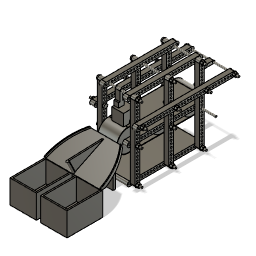
Конвеер v3 (Autodesk Fusion 360 design; units mm, degrees)
Autodesk Fusion 360 part; units mm, degrees
note: some values were not read from the file. Set by a fixed rule: which sketch regions a step uses.
box "BoxPrimitive1" add length 25 width 25 height 25 placed x (0, 0, 1) y (1, 0, 0) z (0, 1, 0) at (0, 0, 0) makes body 1
sketch "Sketch2" plane through (0, 0, 0) normal (0, 1, 0) x (1, 0, 0)
  line L0 (0, 0) -> (-70, 0)
  line L1 (-70, 0) -> (-70, -50)
  line L2 (-70, -50) -> (0, -50)
  line L3 (0, -50) -> (0, 0)
  line L4 (-75, -55) -> (5, -55)
  line L5 (5, -55) -> (5, 5)
  line L6 (5, 5) -> (-75, 5)
  line L7 (-75, 5) -> (-75, -55)
  dimension "d6" = 5
  constraint horizontal L0
  constraint vertical L1
  constraint horizontal L2
  constraint vertical L3
  constraint coincident L0.start L3.end
extrude "Extrude1" add sketch "Sketch2" along normal blind 4 separate body contours L0 L1 L2 L3 makes body 2
extrude "Extrude2" add sketch "Sketch2" along normal blind 50 bodies 2
sketch "Sketch3" plane through (0, 50, 0) normal (0, 1, 0) x (-1, 0, 0)
  line L0 (0, 0) -> (0, 50)
  line L1 (0, 50) -> (70, 50)
  line L2 (70, 50) -> (70, 0)
  line L3 (70, 0) -> (0, 0)
  line L4 (75, -5) -> (75, 55)
  line L5 (75, 55) -> (-5, 55)
  line L6 (-5, 55) -> (-5, -5)
  line L7 (-5, -5) -> (75, -5)
  line L8 (-3, 53) -> (73, 53)
  line L9 (73, 53) -> (73, -3)
  line L10 (73, -3) -> (-3, -3)
  line L11 (-3, -3) -> (-3, 53)
  dimension "d11" = -3
extrude "Extrude3" cut sketch "Sketch3" against normal blind 80 contours L4 L5 L6 L7 bodies 2
sketch "Sketch4" plane through (0, 0, 0) normal (1, 0, 0) x (0, 0, -1)
  line L0 (0, 0) -> (150, 0)
  line L1 (150, 10) -> (0, 10)
  arc A0 (150, 0) -> (150, 10) centre (150, 5) ccw
  arc A1 (0, 10) -> (0, 0) centre (0, 5) ccw
  circle A2 centre (150, 5) radius 2
  circle A3 centre (143.4783, 5) radius 2
  circle A4 centre (136.9565, 5) radius 2
  circle A5 centre (130.4348, 5) radius 2
  circle A6 centre (123.913, 5) radius 2
  circle A7 centre (117.3913, 5) radius 2
  circle A8 centre (110.8696, 5) radius 2
  circle A9 centre (104.3478, 5) radius 2
  circle A10 centre (97.8261, 5) radius 2
  circle A11 centre (91.3043, 5) radius 2
  circle A12 centre (84.7826, 5) radius 2
  circle A13 centre (78.2609, 5) radius 2
  circle A14 centre (71.7391, 5) radius 2
  circle A15 centre (65.2174, 5) radius 2
  circle A16 centre (58.6957, 5) radius 2
  circle A17 centre (52.1739, 5) radius 2
  circle A18 centre (45.6522, 5) radius 2
  circle A19 centre (39.1304, 5) radius 2
  circle A20 centre (32.6087, 5) radius 2
  circle A21 centre (26.087, 5) radius 2
  circle A22 centre (19.5652, 5) radius 2
  circle A23 centre (13.0435, 5) radius 2
  circle A24 centre (6.5217, 5) radius 2
  circle A25 centre (0, 5) radius 2
  dimension "d14" = 4
  dimension "d17" = -150
  dimension "d18" = 0
  constraint horizontal L0
  constraint horizontal L1
  constraint coincident L0.start A1.end
  constraint concentric A0 A2
  measures "d14" diameter of A2
extrude "Extrude4" add sketch "Sketch4" along normal blind 10 separate body makes body 3
sketch "Sketch5" plane through (0, 0, 0) normal (1, 0, 0) x (0, 0, -1)
  circle A0 centre (97.8261, 5) radius 2
  circle A1 centre (26.087, 5) radius 2
  circle A2 centre (32.6087, 5) radius 2
  circle A3 centre (0, 5) radius 2
  circle A4 centre (6.5217, 5) radius 2
  circle A5 centre (13.0435, 5) radius 2
  circle A6 centre (19.5652, 5) radius 2
  circle A7 centre (39.1304, 5) radius 2
  circle A8 centre (65.2174, 5) radius 2
  circle A9 centre (45.6522, 5) radius 2
  circle A10 centre (52.1739, 5) radius 2
  circle A11 centre (71.7391, 5) radius 2
  circle A12 centre (91.3043, 5) radius 2
  circle A13 centre (84.7826, 5) radius 2
  circle A14 centre (78.2609, 5) radius 2
  circle A15 centre (58.6957, 5) radius 2
  circle A16 centre (150, 5) radius 2
  circle A17 centre (136.9565, 5) radius 2
  circle A18 centre (143.4783, 5) radius 2
  circle A19 centre (130.4348, 5) radius 2
  circle A20 centre (110.8696, 5) radius 2
  circle A21 centre (104.3478, 5) radius 2
  circle A22 centre (117.3913, 5) radius 2
  circle A23 centre (123.913, 5) radius 2
  arc A24 (0, 10) -> (0, 0) centre (0, 5) ccw
  line L0 (0, 10) -> (150, 10)
  arc A25 (150, 0) -> (150, 10) centre (150, 5) ccw
  line L1 (150, 0) -> (0, 0)
  circle A26 centre (143.4783, 5) radius 20
  circle A27 centre (143.4783, 5) radius 23
  dimension "d21" = 40
  dimension "d22" = 46
  constraint concentric A18 A26
  constraint concentric A18 A27
  measures "d21" diameter of A26
  measures "d22" diameter of A27
extrude "Extrude5" add sketch "Sketch5" against normal blind 40 separate body contours A16 | A17 | A19 | A23 A26 | A23 L0 A25 L1 A26 | A23 A26 | A23 L0 L1 A26 A27 | L0 A25 L1 A26 | L0 L1 A26 A27 makes body 4
copy_body "CopyPasteBodies1" bodies 3 makes body 5
move_body "Move1" bodies 5 to x (1, 0, 0) y (0, 1, 0) z (0, 0, 1) at (-50, 0, 0)
copy_body "CopyPasteBodies2" bodies 4 makes body 6
move_body "Move2" bodies 6 to x (1, 0, 0) y (0, 1, 0) z (0, 0, 1) at (0, 0, 137)
copy_body "CopyPasteBodies3" bodies 4 makes body 7
move_body "Move3" bodies 7 to x (1, 0, 0) y (0, 1, 0) z (0, 0, 1) at (0, 0, 65)
move_body "Align1" bodies 7 to x (1, 0, 0) y (0, 1, 0) z (0, 0, 1) at (0, 0, 0.2174)
sketch "Sketch6" plane through (-40, 0, 0) normal (-1, 0, 0) x (0, 0, 1)
  circle A0 centre (-143.4783, 5) radius 2
  circle A1 centre (-143.4783, 5) radius 23
  circle A2 centre (-143.4783, 5) radius 23
  circle A3 centre (-78.2609, 5) radius 23
  circle A4 centre (-6.4783, 5) radius 23
  line L0 (-6.4783, 5) -> (-6.4783, 28)
  line L1 (-143.4783, 5) -> (-143.4783, 28)
  line L2 (-143.4783, 28) -> (-6.4783, 28)
  line L3 (-143.4783, 5) -> (-143.4783, -18)
  line L4 (-6.4783, 5) -> (-6.4783, -18)
  line L5 (-6.4783, -18) -> (-143.4783, -18)
  arc A5 (-143.4783, 28) -> (-143.4783, -18) centre (-143.4783, 5) ccw
  arc A6 (-6.4783, -18) -> (-6.4783, 28) centre (-6.4783, 5) ccw
  arc A7 (-143.4783, 29) -> (-143.4783, -19) centre (-143.4783, 5) ccw
  line L6 (-6.4783, -19) -> (-143.4783, -19)
  arc A8 (-6.4783, -19) -> (-6.4783, 29) centre (-6.4783, 5) ccw
  line L7 (-143.4783, 29) -> (-6.4783, 29)
  dimension "d25" = 1
  constraint coincident A4.centre L0.start
  constraint coincident A4 L0.end
  constraint vertical L0
  constraint coincident A0.centre A1.centre
  constraint coincident A2 L1.end
  constraint parallel L0 L1
  constraint coincident A2 L3.end
  constraint perpendicular L2 L3
  constraint coincident A4 L4.end
  constraint parallel L0 L4
  constraint tangent L5 A5
  constraint tangent L2 A6
extrude "Extrude6" add sketch "Sketch6" against normal blind 40 separate body makes body 8
sketch "Sketch7" plane through (0, 0, 0) normal (1, 0, 0) x (0, 0, -1)
  arc A0 (6.4783, 29) -> (6.4783, -19) centre (6.4783, 5) ccw
  line L0 (-20, -19) -> (-90, -19)
  line L1 (-20, 15) -> (-20, -19)
  line L2 (-20, 15) -> (-90, -19)
  constraint tangent A0 L0
  constraint perpendicular L0 L1
extrude "Extrude7" add sketch "Sketch7" against normal blind 40 separate body makes body 9
move_body "Move4" bodies 2 to x (0, 0, -1) y (0, 1, 0) z (1, 0, 0) at (-70, -71, 89)
move_body "Move5" bodies 2 to x (1, 0, 0) y (0, 1, 0) z (0, 0, 1) at (25, 0, 0)
copy_body "CopyPasteBodies4" bodies 5 makes body 10
move_body "Move6" bodies 10 to x (1, 0, 0) y (0, 1, 0) z (0, 0, 1) at (0, -72, 0)
sketch "Sketch8" plane through (-50, 0, 0) normal (-1, 0, 0) x (0, 0, 1)
  circle A0 centre (-97.8261, -67) radius 2
  circle A1 centre (-26.087, -67) radius 2
  circle A2 centre (-32.6087, -67) radius 2
  circle A3 centre (0, -67) radius 2
  circle A4 centre (-6.5217, -67) radius 2
  circle A5 centre (-13.0435, -67) radius 2
  circle A6 centre (-19.5652, -67) radius 2
  circle A7 centre (-39.1304, -67) radius 2
  circle A8 centre (-65.2174, -67) radius 2
  circle A9 centre (-45.6522, -67) radius 2
  circle A10 centre (-52.1739, -67) radius 2
  circle A11 centre (-71.7391, -67) radius 2
  circle A12 centre (-91.3043, -67) radius 2
  circle A13 centre (-84.7826, -67) radius 2
  circle A14 centre (-78.2609, -67) radius 2
  circle A15 centre (-58.6957, -67) radius 2
  circle A16 centre (-150, -67) radius 2
  circle A17 centre (-136.9565, -67) radius 2
  circle A18 centre (-143.4783, -67) radius 2
  circle A19 centre (-130.4348, -67) radius 2
  circle A20 centre (-110.8696, -67) radius 2
  circle A21 centre (-104.3478, -67) radius 2
  circle A22 centre (-117.3913, -67) radius 2
  circle A23 centre (-123.913, -67) radius 2
  arc A24 (0, -72) -> (0, -62) centre (0, -67) ccw
  line L0 (0, -62) -> (-150, -62)
  arc A25 (-150, -62) -> (-150, -72) centre (-150, -67) ccw
  line L1 (-150, -72) -> (0, -72)
  line L2 (-136.9565, -67) -> (-141.9565, -67)
  line L3 (-136.9565, -67) -> (-131.9565, -67)
  arc A26 (-141.9565, -67) -> (-131.9565, -67) centre (-136.9565, -67) ccw
  circle A27 centre (-136.9565, -67) radius 2
  line L4 (-141.9565, -67) -> (-141.9565, 90)
  line L5 (-131.9565, -67) -> (-131.9565, -62)
  line L6 (-131.9565, 90) -> (-131.9565, -62)
  arc A28 (-131.9565, 90) -> (-141.9565, 90) centre (-136.9565, 90) ccw
  circle A29 centre (-136.9565, -60.4583) radius 2
  circle A30 centre (-136.9565, -53.9167) radius 2
  circle A31 centre (-136.9565, -47.375) radius 2
  circle A32 centre (-136.9565, -40.8333) radius 2
  circle A33 centre (-136.9565, -34.2917) radius 2
  circle A34 centre (-136.9565, -27.75) radius 2
  circle A35 centre (-136.9565, -21.2083) radius 2
  circle A36 centre (-136.9565, -14.6667) radius 2
  circle A37 centre (-136.9565, -8.125) radius 2
  circle A38 centre (-136.9565, -1.5833) radius 2
  circle A39 centre (-136.9565, 4.9583) radius 2
  circle A40 centre (-136.9565, 11.5) radius 2
  circle A41 centre (-136.9565, 18.0417) radius 2
  circle A42 centre (-136.9565, 24.5833) radius 2
  circle A43 centre (-136.9565, 31.125) radius 2
  circle A44 centre (-136.9565, 37.6667) radius 2
  circle A45 centre (-136.9565, 44.2083) radius 2
  circle A46 centre (-136.9565, 50.75) radius 2
  circle A47 centre (-136.9565, 57.2917) radius 2
  circle A48 centre (-136.9565, 63.8333) radius 2
  circle A49 centre (-136.9565, 70.375) radius 2
  circle A50 centre (-136.9565, 76.9167) radius 2
  circle A51 centre (-136.9565, 83.4583) radius 2
  circle A52 centre (-136.9565, 90) radius 2
  dimension "d30" = 10
  dimension "d33" = 0
  dimension "d34" = 157
  constraint concentric A17 A26
  constraint tangent L1 A26
  constraint coincident A17.centre L2.start
  constraint horizontal L2
  constraint parallel L2 L3
  constraint tangent A26 L4
  constraint tangent A26 L5
  constraint coincident L0 L5.end
  measures "d30" distance of L4.end L6.start
extrude "Extrude8" add sketch "Sketch8" along normal blind 10 separate body contours A17 A18 A19 L2 L3 A26 A27 | A17 A18 A19 L0 L2 L3 A27 L4 L5 A29 | A19 L3 A26 | A19 L3 L5 | A18 L2 L4 | A18 L2 A26 | L0 L4 L6 A28 A29 makes body 11
copy_body "CopyPasteBodies5" bodies 11 makes body 12
move_body "Move7" bodies 12 to x (1, 0, 0) y (0, 1, 0) z (0, 0, 1) at (0, 0, 131)
move_body "Move8" bodies 12 to x (1, 0, 0) y (0, 1, 0) z (0, 0, 1) at (-50, 0, 0)
move_body "Align2" bodies 12 to x (1, 0, 0) y (0, 1, 0) z (0, 0, 1) at (50, 0, -0.5652)
copy_body "CopyPasteBodies6" bodies 12 makes body 13
move_body "Move9" bodies 13 to x (1, 0, 0) y (0, 1, 0) z (0, 0, 1) at (-56, 0, -72)
move_body "Align3" bodies 13 to x (1, 0, 0) y (0, 1, 0) z (0, 0, 1) at (56, 0, 0.2609)
extrude "Extrude9" add 1 faces at (-40, -71, -73.913) along direction (1, 0, 0) blind 50 separate body on bodies 10 makes body 14
combine "Combine1" operation add target body 14 tool bodies 10
copy_body "CopyPasteBodies7" bodies 13 12 11 makes body 15 makes body 16 makes body 17
move_body "Move10" bodies 15 16 17 to x (1, 0, 0) y (0, 1, 0) z (0, 0, 1) at (70, 0, 0)
copy_body "CopyPasteBodies8" bodies 3 5 makes body 18 makes body 19
move_body "Move11" bodies 18 19 to x (1, 0, 0) y (0, 1, 0) z (0, 0, 1) at (0, 85, 0)
sketch "Sketch9" plane through (-40, 0, 0) normal (-1, 0, 0) x (0, 0, 1)
  line L0 (20, 15) -> (20, -19)
  line L1 (20, -19) -> (90, -19)
  line L2 (90, -19) -> (20, 15)
  line L3 (20, 15) -> (90, -19)
  line L4 (90, -19) -> (103.0246, 7.8154)
  line L5 (103.0246, 7.8154) -> (29.3484, 10.4593)
  constraint coincident L0.start L2.end
  constraint coincident L1.end L2.start
  constraint perpendicular L3 L4
  constraint coincident L2 L5.end
extrude "Extrude10" add sketch "Sketch9" against normal blind 3 separate body contours L2 L3 L4 L5 makes body 20
move_body "Move12" bodies 20 to x (1, 0, 0) y (0, 1, 0) z (0, 0, 1) at (17, 0, 0)
move_body "Move13" bodies 16 to x (1, 0, 0) y (0, 1, 0) z (0, 0, 1) at (60, 0, 0)
move_body "Move14" bodies 15 to x (1, 0, 0) y (0, 1, 0) z (0, 0, 1) at (60, 0, 0)
move_body "Align4" bodies 16 to x (1, 0, 0) y (0, 1, 0) z (0, 0, 1) at (-60, 0, 6.5217)
move_body "Align5" bodies 15 to x (1, 0, 0) y (0, 1, 0) z (0, 0, 1) at (-60, 0, 0)
move_body "Move15" bodies 16 to x (1, 0, 0) y (0, 1, 0) z (0, 0, 1) at (50, 0, 0)
move_body "Align6" bodies 16 to x (1, 0, 0) y (0, 1, 0) z (0, 0, 1) at (-50, 0, -6.5217)
sketch "Sketch10" plane through (20, 0, 0) normal (1, 0, 0) x (0, 0, -1)
  circle A0 centre (6.5217, 50.75) radius 2
  circle A1 centre (6.5217, 57.2917) radius 2
  circle A2 centre (6.5217, 63.8333) radius 2
  circle A3 centre (6.5217, 76.9167) radius 2
  circle A4 centre (6.5217, 4.9583) radius 2
  circle A5 centre (6.5217, 70.375) radius 2
  circle A6 centre (6.5217, 11.5) radius 2
  circle A7 centre (6.5217, 44.2083) radius 2
  circle A8 centre (6.5217, 24.5833) radius 2
  circle A9 centre (6.5217, 31.125) radius 2
  circle A10 centre (6.5217, 37.6667) radius 2
  circle A11 centre (6.5217, 18.0417) radius 2
  circle A12 centre (6.5217, -40.8333) radius 2
  circle A13 centre (6.5217, -47.375) radius 2
  circle A14 centre (6.5217, -53.9167) radius 2
  circle A15 centre (6.5217, -1.5833) radius 2
  circle A16 centre (6.5217, -34.2917) radius 2
  circle A17 centre (6.5217, -27.75) radius 2
  circle A18 centre (6.5217, -21.2083) radius 2
  circle A19 centre (6.5217, -8.125) radius 2
  circle A20 centre (6.5217, -14.6667) radius 2
  circle A21 centre (6.5217, -60.4583) radius 2
  circle A22 centre (6.5217, 83.4583) radius 2
  circle A23 centre (6.5217, -67) radius 2
  circle A24 centre (6.5217, 90) radius 2
  arc A25 (1.5217, -67) -> (11.5217, -67) centre (6.5217, -67) ccw
  line L0 (11.5217, -67) -> (11.5217, 90)
  arc A26 (11.5217, 90) -> (1.5217, 90) centre (6.5217, 90) ccw
  line L1 (1.5217, 90) -> (1.5217, -67)
move_body "Move16" bodies 5 to x (1, 0, 0) y (0, 1, 0) z (0, 0, 1) at (20, 0, 0)
move_body "Align7" bodies 5 to x (1, 0, 0) y (0, 1, 0) z (0, 0, 1) at (-20, -0.0417, 0)
move_body "Move17" bodies 3 to x (1, 0, 0) y (0, 1, 0) z (0, 0, 1) at (-15, 0, 0)
move_body "Align8" bodies 3 to x (1, 0, 0) y (0, 1, 0) z (0, 0, 1) at (15, -0.0417, 0)
move_body "Align9" bodies 5 to x (1, 0, 0) y (0, 1, 0) z (0, 0, 1) at (0, 0.0417, 0.0435)
sketch "Sketch11" plane through (-60, 0, 0) normal (-1, 0, 0) x (0, 0, 1)
  circle A0 centre (-136.9565, 50.75) radius 2
  circle A1 centre (-136.9565, 57.2917) radius 2
  circle A2 centre (-136.9565, 63.8333) radius 2
  circle A3 centre (-136.9565, 76.9167) radius 2
  circle A4 centre (-136.9565, 4.9583) radius 2
  circle A5 centre (-136.9565, 70.375) radius 2
  circle A6 centre (-136.9565, 11.5) radius 2
  circle A7 centre (-136.9565, 44.2083) radius 2
  circle A8 centre (-136.9565, 24.5833) radius 2
  circle A9 centre (-136.9565, 31.125) radius 2
  circle A10 centre (-136.9565, 37.6667) radius 2
  circle A11 centre (-136.9565, 18.0417) radius 2
  circle A12 centre (-136.9565, -40.8333) radius 2
  circle A13 centre (-136.9565, -47.375) radius 2
  circle A14 centre (-136.9565, -53.9167) radius 2
  circle A15 centre (-136.9565, -1.5833) radius 2
  circle A16 centre (-136.9565, -34.2917) radius 2
  circle A17 centre (-136.9565, -27.75) radius 2
  circle A18 centre (-136.9565, -21.2083) radius 2
  circle A19 centre (-136.9565, -8.125) radius 2
  circle A20 centre (-136.9565, -14.6667) radius 2
  circle A21 centre (-136.9565, -60.4583) radius 2
  circle A22 centre (-136.9565, 83.4583) radius 2
  circle A23 centre (-136.9565, -67) radius 2
  circle A24 centre (-136.9565, 90) radius 2
  arc A25 (-141.9565, -67) -> (-131.9565, -67) centre (-136.9565, -67) ccw
  line L0 (-131.9565, -67) -> (-131.9565, 90)
  arc A26 (-131.9565, 90) -> (-141.9565, 90) centre (-136.9565, 90) ccw
  line L1 (-141.9565, 90) -> (-141.9565, -67)
  circle A27 centre (-136.9565, 90) radius 4
  dimension "d41" = 8
  constraint concentric A24 A27
  measures "d41" diameter of A27
extrude "Extrude11" add sketch "Sketch11" against normal blind 90 separate body contours A24 makes body 21
extrude "Extrude12" add sketch "Sketch11" along normal blind 3 separate body contours A24 | A27 makes body 22
combine "Combine2" operation add target body 22 tool bodies 21
copy_body "CopyPasteBodies9" bodies 22 makes body 23
copy_body "CopyPasteBodies10" bodies 23 makes body 24
sketch "Sketch12" plane through (20, 0, 0) normal (1, 0, 0) x (0, 0, -1)
  circle A0 centre (136.9565, 50.75) radius 2
  circle A1 centre (136.9565, 57.2917) radius 2
  circle A2 centre (136.9565, 63.8333) radius 2
  circle A3 centre (136.9565, 76.9167) radius 2
  circle A4 centre (136.9565, 4.9583) radius 2
  circle A5 centre (136.9565, 70.375) radius 2
  circle A6 centre (136.9565, 11.5) radius 2
  circle A7 centre (136.9565, 44.2083) radius 2
  circle A8 centre (136.9565, 24.5833) radius 2
  circle A9 centre (136.9565, 31.125) radius 2
  circle A10 centre (136.9565, 37.6667) radius 2
  circle A11 centre (136.9565, 18.0417) radius 2
  circle A12 centre (136.9565, -40.8333) radius 2
  circle A13 centre (136.9565, -47.375) radius 2
  circle A14 centre (136.9565, -53.9167) radius 2
  circle A15 centre (136.9565, -1.5833) radius 2
  circle A16 centre (136.9565, -34.2917) radius 2
  circle A17 centre (136.9565, -27.75) radius 2
  circle A18 centre (136.9565, -21.2083) radius 2
  circle A19 centre (136.9565, -8.125) radius 2
  circle A20 centre (136.9565, -14.6667) radius 2
  circle A21 centre (136.9565, -60.4583) radius 2
  circle A22 centre (136.9565, 83.4583) radius 2
  circle A23 centre (136.9565, -67) radius 2
  circle A24 centre (136.9565, 90) radius 2
  arc A25 (131.9565, -67) -> (141.9565, -67) centre (136.9565, -67) ccw
  line L0 (141.9565, -67) -> (141.9565, 90)
  arc A26 (141.9565, 90) -> (131.9565, 90) centre (136.9565, 90) ccw
  line L1 (131.9565, 90) -> (131.9565, -67)
  circle A27 centre (136.9565, 90) radius 2
  line L2 (134.9358, 93.5) -> (132.9151, 90)
  line L3 (132.9151, 90) -> (134.9358, 86.5)
  line L4 (134.9358, 86.5) -> (138.9772, 86.5)
  line L5 (138.9772, 86.5) -> (140.998, 90)
  line L6 (140.998, 90) -> (138.9772, 93.5)
  line L7 (138.9772, 93.5) -> (134.9358, 93.5)
  point P0 (136.9565, 90)
  dimension "d46" = 3.5
  constraint coincident P0 A24.centre
  measures "d46" distance of P0 L7
extrude "Extrude13" add sketch "Sketch12" along normal blind 5 separate body contours L2 L3 L4 L5 L6 L7 makes body 25
copy_body "CopyPasteBodies11" bodies 25 24 makes body 26 makes body 27
move_body "Move18" bodies 26 27 to x (1, 0, 0) y (0, 1, 0) z (0, 0, 1) at (0, 0, 59)
copy_body "CopyPasteBodies12" bodies 27 26 makes body 28 makes body 29
move_body "Move19" bodies 28 29 to x (1, 0, 0) y (0, 1, 0) z (0, 0, 1) at (0, 0, 70)
delete_body "RemoveBody2" bodies 23
delete_body "RemoveBody3" bodies 22
move_body "Align10" bodies 17 to x (1, 0, 0) y (0, 1, 0) z (0, 0, 1) at (0, 0, 0)
move_body "Align11" bodies 27 to x (1, 0, 0) y (0, 1, 0) z (0, 0, 1) at (0, 0, -0.3043)
move_body "Align12" bodies 28 to x (1, 0, 0) y (0, 1, 0) z (0, 0, 1) at (0, 0, 1.4348)
move_body "Align13" bodies 26 to x (0, 0, 1) y (0, 1, 0) z (-1, 0, 0) at (-55.4565, 0, -100.7609)
move_body "Align14" bodies 26 to x (0, 0, 1) y (0, 1, 0) z (-1, 0, 0) at (-53.2609, 0, -100.7609)
move_body "Move20" bodies 26 to x (1, 0, 0) y (0, 1, 0) z (0, 0, 1) at (5.5, 0, 0)
move_body "Align15" bodies 26 to x (1, 0, 0) y (0, 1, 0) z (0, 0, 1) at (-8, 0, 0)
move_body "Align16" bodies 29 to x (1, 0, 0) y (0, 1, 0) z (0, 0, 1) at (0, 0, 1.4348)
copy_body "CopyPasteBodies13" bodies 29 28 27 26 25 24 makes body 30 makes body 31 makes body 32 makes body 33 makes body 34 makes body 35
move_body "Move21" bodies 30 31 32 33 34 35 to x (1, 0, 0) y (0, 1, 0) z (0, 0, 1) at (0, -85, 0)
move_body "Align17" bodies 11 to x (1, 0, 0) y (0, 1, 0) z (0, 0, 1) at (0, 0, -6.5217)
move_body "Align18" bodies 17 to x (1, 0, 0) y (0, 1, 0) z (0, 0, 1) at (0, 0, -6.5217)
move_body "Align19" bodies 24 to x (1, 0, 0) y (0, 1, 0) z (0, 0, 1) at (0, 0, -6.5217)
move_body "Align20" bodies 25 to x (1, 0, 0) y (0, 1, 0) z (0, 0, 1) at (0, 0, -6.5217)
move_body "Align21" bodies 35 to x (1, 0, 0) y (0, 1, 0) z (0, 0, 1) at (0, -0.0417, -6.5217)
move_body "Align22" bodies 34 to x (1, 0, 0) y (0, 1, 0) z (0, 0, 1) at (0, -0.0417, -6.5217)
copy_body "CopyPasteBodies14" bodies 35 34 33 32 31 30 makes body 36 makes body 37 makes body 38 makes body 39 makes body 40 makes body 41
move_body "Move22" bodies 36 37 38 39 40 41 to x (1, 0, 0) y (0, 1, 0) z (0, 0, 1) at (0, -72, 0)
move_body "Move23" bodies 20 to x (1, 0, 0) y (0, 1, 0) z (0, 0, 1) at (0, 2.1845, -4.4975)
sketch "Sketch13" plane through (0, 19.9967, 9.7127) normal (0, 0.899508, 0.436904) x (1, 0, 0)
  line L0 (0, -89.2569) -> (0, -11.4366)
  line L1 (0, -11.4366) -> (-40, -11.4366)
  line L2 (-40, -11.4366) -> (-40, -89.2569)
  line L3 (-40, -89.2569) -> (0, -89.2569)
  line L4 (-23, -16.8294) -> (-23, -84.2569)
  line L5 (-23, -84.2569) -> (-20, -84.2569)
  line L6 (-20, -84.2569) -> (-20, -16.8294)
  line L7 (-20, -16.8294) -> (-23, -16.8294)
  line L8 (-23, -84.2569) -> (-23.7059, -85.5804)
  line L9 (-20, -84.2569) -> (-19.2941, -85.5804)
  arc A0 (-23.7059, -85.5804) -> (-19.2941, -85.5804) centre (-21.5, -86.7569) ccw
  constraint tangent L5 A0
  constraint coincident L4.end L5.start
  constraint tangent L8 A0
  constraint coincident L5.end L6.start
  constraint tangent L9 A0
extrude "Extrude14" add sketch "Sketch13" along normal blind 29.9 separate body contours L5 L8 L9 A0 makes body 42
combine "Combine3" operation add target body 20 tool bodies 42
copy_body "CopyPasteBodies15" bodies 2 makes body 43
move_body "Move24" bodies 43 to x (1, 0, 0) y (0, 1, 0) z (0, 0, 1) at (-65, 0, 0)
move_body "Move25" bodies 2 43 to x (1, 0, 0) y (0, 1, 0) z (0, 0, 1) at (31, 0, 0)
sketch "Sketch14" plane through (-40, 0, 0) normal (-1, 0, 0) x (0, 0, 1)
  line L0 (20, 15) -> (20, -19)
  line L1 (20, -19) -> (90, -19)
  line L2 (90, -19) -> (20, 15)
  circle A0 centre (-97.8261, -67) radius 2
  circle A1 centre (-26.087, -67) radius 2
  circle A2 centre (-32.6087, -67) radius 2
  circle A3 centre (0, -67) radius 2
  circle A4 centre (-6.5217, -67) radius 2
  circle A5 centre (-13.0435, -67) radius 2
  circle A6 centre (-19.5652, -67) radius 2
  circle A7 centre (-39.1304, -67) radius 2
  circle A8 centre (-65.2174, -67) radius 2
  circle A9 centre (-45.6522, -67) radius 2
  circle A10 centre (-52.1739, -67) radius 2
  circle A11 centre (-71.7391, -67) radius 2
  circle A12 centre (-91.3043, -67) radius 2
  circle A13 centre (-84.7826, -67) radius 2
  circle A14 centre (-78.2609, -67) radius 2
  circle A15 centre (-58.6957, -67) radius 2
  circle A16 centre (-150, -67) radius 2
  circle A17 centre (-136.9565, -67) radius 2
  circle A18 centre (-143.4783, -67) radius 2
  circle A19 centre (-130.4348, -67) radius 2
  circle A20 centre (-110.8696, -67) radius 2
  circle A21 centre (-104.3478, -67) radius 2
  circle A22 centre (-117.3913, -67) radius 2
  circle A23 centre (-123.913, -67) radius 2
  arc A24 (0, -72) -> (0, -62) centre (0, -67) ccw
  line L3 (0, -62) -> (-150, -62)
  arc A25 (-150, -62) -> (-150, -72) centre (-150, -67) ccw
  line L4 (-150, -72) -> (0, -72)
  line L5 (0, -72) -> (85, -72)
  line L6 (20, -19) -> (20, -72)
  line L7 (20, -72) -> (25, -72)
  line L8 (25, -72) -> (25, -19)
  line L9 (25, -19) -> (70, -19)
  line L10 (70, -19) -> (70, -72)
  line L11 (70, -72) -> (75, -72)
  line L12 (75, -72) -> (75, -19)
  dimension "d51" = 5
  constraint coincident A24.start L4.end
  constraint tangent A24 L5
  constraint coincident L0.end L1.start
  constraint coincident L5 L6.end
  constraint perpendicular L5 L6
  constraint perpendicular L6 L7
  constraint coincident L1 L8.end
  constraint perpendicular L1 L8
  constraint coincident L1 L9.end
  constraint coincident L5 L10.end
  constraint perpendicular L5 L10
  constraint coincident L5 L11.end
  constraint coincident L1 L12.end
  constraint perpendicular L1 L12
  measures "d51" distance of L6.end L7.end
extrude "Extrude15" add sketch "Sketch14" against normal blind 40 separate body contours L1 L5 L6 L7 L8 | L1 L5 L10 L11 L12 makes body 44 at (-26.6667, -54.3333, 25) makes body 45 at (-26.6667, -54.3333, 75)
combine "Combine4" operation add target body 45 tool bodies 44 9
sketch "Sketch15" plane through (0, 0, 0) normal (1, 0, 0) x (0, 0, -1)
  line L0 (-70, -72) -> (-70, -19)
  line L1 (-70, -19) -> (-25, -19)
  line L2 (-25, -19) -> (-25, -72)
  line L3 (-25, -72) -> (-20, -72)
  line L4 (-20, -72) -> (-20, 15)
  line L5 (-20, 15) -> (-90, -19)
  line L6 (-90, -19) -> (-75, -19)
  line L7 (-75, -19) -> (-75, -72)
  line L8 (-75, -72) -> (-70, -72)
  line L9 (-20, 15) -> (-20, 11)
  line L10 (-90, -19) -> (-90, -23)
  line L11 (-90, -23) -> (-20, 11)
  constraint coincident L4.end L5.start
  constraint coincident L4 L9.end
  constraint parallel L4 L9
  constraint coincident L5.end L6.start
  constraint perpendicular L6 L10
extrude "Extrude16" add sketch "Sketch15" along normal blind 40 separate body contours L4 L5 L6 L9 L11 makes body 46
copy_body "CopyPasteBodies16" bodies 46 makes body 47
move_body "Move26" bodies 47 to x (1, 0, 0) y (0, 1, 0) z (0, 0, 1) at (-80, 0, 0)
combine "Combine5" operation add target body 47 tool bodies 45 46
sketch "Sketch16" plane through (0, 19.9967, 9.7127) normal (0, 0.899508, 0.436904) x (1, 0, 0)
  line L0 (-80, -11.4366) -> (-80, -89.2569)
  line L1 (-80, -89.2569) -> (40, -89.2569)
  line L2 (40, -89.2569) -> (40, -11.4366)
  line L3 (40, -11.4366) -> (-80, -11.4366)
  arc A0 (-53.5072, -11.4366) -> (-80, -89.2569) centre (47.5418, -89.2569) ccw
  line L4 (-23, -16.8294) -> (-20, -16.8294)
  line L5 (-20, -89.2569) -> (-20, -80)
  arc A1 (40, -89.2569) -> (13.5072, -11.4366) centre (-87.5418, -89.2569) ccw
  constraint tangent L0 A0
  constraint coincident L3 A0.start
  constraint coincident L0.end L1.start
  constraint midpoint L1 L5.start
  constraint perpendicular L1 L5
  constraint symmetric L0.end L5 L1.end
  constraint symmetric A0.start L5 A1.end
  constraint symmetric A0 L5 A1
extrude "Extrude17" cut sketch "Sketch16" against normal blind 5 contours L0 L3 A0 | L2 L3 A1 bodies 43 47
sketch "Sketch17" plane through (0, 19.9967, 9.7127) normal (0, 0.899508, 0.436904) x (1, 0, 0)
  arc A0 (-53.5072, -11.4366) -> (-80, -89.2569) centre (47.5418, -89.2569) ccw
  line L0 (-80, -89.2569) -> (40, -89.2569)
  arc A1 (40, -89.2569) -> (13.5072, -11.4366) centre (-87.5418, -89.2569) ccw
  line L1 (13.5072, -11.4366) -> (-53.5072, -11.4366)
  line L2 (-80, -89.2569) -> (-78, -89.2569)
  line L3 (40, -89.2569) -> (38, -89.2569)
  line L4 (13.5072, -11.4366) -> (11.5072, -11.4366)
  line L5 (-53.5072, -11.4366) -> (-51.5072, -11.4366)
  arc A2 (-51.5072, -11.4366) -> (-78, -89.2569) centre (48.5107, -88.9059) ccw
  arc A3 (38, -89.2569) -> (11.5072, -11.4366) centre (-88.5107, -88.9059) ccw
  dimension "d58" = 2
  dimension "d59" = 2
  dimension "d60" = 2
  constraint coincident A0.end L0.start
  constraint parallel L0 L2
  constraint coincident L0.end A1.start
  constraint coincident L0 L3.end
  constraint parallel L0 L3
  constraint coincident A1.end L1.start
  constraint parallel L1 L4
  constraint coincident A0.start L1.end
  constraint parallel L1 L5
  constraint tangent A0 A2
  constraint tangent A1 A3
  measures "d58" distance of A0.end L2.end
  measures "d59" distance of A1.end L4.end
  measures "d60" distance of A0.start L5.end
extrude "Extrude18" add sketch "Sketch17" along normal blind 4 separate body contours A0 L0 L1 L2 L5 A2 | L0 A1 L1 L3 L4 A3 makes body 48 at (-76.0966, -6.8948, 71.1811) makes body 49 at (37.5387, -11.7297, 81.1353)
combine "Combine6" operation add target body 49 tool bodies 47 48
sketch "Sketch18" plane through (30, 0, 0) normal (1, 0, 0) x (0, 0, -1)
  circle A0 centre (6.5217, 90) radius 2
  circle A1 centre (6.5217, 90) radius 3
  line L0 (6.5217, 90) -> (3.5217, 90)
  line L1 (6.5217, 90) -> (9.5217, 90)
  line L2 (9.5217, 90) -> (9.5217, 70)
  line L3 (9.5217, 70) -> (3.5217, 70)
  line L4 (3.5217, 70) -> (3.5217, 90)
  line L5 (9.5217, 70) -> (12.5217, 70)
  line L6 (12.5217, 70) -> (12.5217, 60)
  line L7 (12.5217, 60) -> (0.5217, 60)
  line L8 (0.5217, 60) -> (0.5217, 70)
  line L9 (0.5217, 70) -> (3.5217, 70)
  dimension "d63" = 6
  dimension "d64" = 3
  dimension "d65" = 10
  dimension "d66" = 12
  constraint concentric A0 A1
  constraint coincident A0.centre A1.centre
  constraint coincident A1 L0.end
  constraint horizontal L0
  constraint coincident A1 L1.end
  constraint parallel L0 L1
  constraint tangent A1 L2
  constraint perpendicular L2 L3
  constraint tangent A1 L4
  constraint perpendicular L2 L5
  constraint perpendicular L5 L6
  constraint perpendicular L4 L7
  constraint perpendicular L7 L8
  constraint perpendicular L8 L9
  measures "d63" diameter of A1
  measures "d64" distance of L2.end L5.end
  measures "d65" distance of L5.end L6.end
  measures "d66" distance of L6.end L7.end
extrude "Extrude19" add sketch "Sketch18" against normal blind 10 separate body contours A0 A1 L0 L1 | A0 A1 L0 L1 | A1 L2 L3 L4 | L3 L5 L6 L7 L8 L9 makes body 50
move_body "Move27" bodies 50 to x (1, 0, 0) y (0, 1, 0) z (0, 0, 1) at (-44, 0, 0)
move_body "Move28" bodies 1 to x (1, 0, 0) y (0, 1, 0) z (0, 0, 1) at (0, 29, -27)
move_body "Move29" bodies 1 to x (1, 0, 0) y (0, 1, 0) z (0, 0, 1) at (-30, 0, 0)
copy_body "CopyPasteBodies17" bodies 3 makes body 51
move_body "Move30" bodies 51 to x (1, 0, 0) y (0, 1, 0) z (0, 0, 1) at (0, 40, 0)
move_body "Align23" bodies 51 to x (1, 0, 0) y (0, 1, 0) z (0, 0, 1) at (0, -0.75, 0)
move_body "Move31" bodies 51 to x (1, 0, 0) y (0, 1, 0) z (0, 0, 1) at (20, 0, 0)
sketch "Sketch19" plane through (30, 0, 0) normal (1, 0, 0) x (0, 0, -1)
  circle A0 centre (97.8261, 44.2083) radius 2
  circle A1 centre (26.087, 44.2083) radius 2
  circle A2 centre (32.6087, 44.2083) radius 2
  circle A3 centre (0, 44.2083) radius 2
  circle A4 centre (6.5217, 44.2083) radius 2
  circle A5 centre (13.0435, 44.2083) radius 2
  circle A6 centre (19.5652, 44.2083) radius 2
  circle A7 centre (39.1304, 44.2083) radius 2
  circle A8 centre (65.2174, 44.2083) radius 2
  circle A9 centre (45.6522, 44.2083) radius 2
  circle A10 centre (52.1739, 44.2083) radius 2
  circle A11 centre (71.7391, 44.2083) radius 2
  circle A12 centre (91.3043, 44.2083) radius 2
  circle A13 centre (84.7826, 44.2083) radius 2
  circle A14 centre (78.2609, 44.2083) radius 2
  circle A15 centre (58.6957, 44.2083) radius 2
  circle A16 centre (150, 44.2083) radius 2
  circle A17 centre (136.9565, 44.2083) radius 2
  circle A18 centre (143.4783, 44.2083) radius 2
  circle A19 centre (130.4348, 44.2083) radius 2
  circle A20 centre (110.8696, 44.2083) radius 2
  circle A21 centre (104.3478, 44.2083) radius 2
  circle A22 centre (117.3913, 44.2083) radius 2
  circle A23 centre (123.913, 44.2083) radius 2
  arc A24 (0, 49.2083) -> (0, 39.2083) centre (0, 44.2083) ccw
  line L0 (0, 39.2083) -> (150, 39.2083)
  arc A25 (150, 39.2083) -> (150, 49.2083) centre (150, 44.2083) ccw
  line L1 (150, 49.2083) -> (0, 49.2083)
  line L2 (150, 44.2083) -> (156.522, 44.2083)
  line L3 (156.522, 44.2083) -> (163.044, 44.2083)
  line L4 (163.044, 44.2083) -> (169.566, 44.2083)
  line L5 (169.566, 44.2083) -> (176.088, 44.2083)
  line L6 (176.088, 44.2083) -> (182.61, 44.2083)
  line L7 (182.61, 44.2083) -> (189.132, 44.2083)
  line L8 (189.132, 44.2083) -> (195.654, 44.2083)
  line L9 (195.654, 44.2083) -> (202.176, 44.2083)
  circle A26 centre (156.522, 44.2083) radius 2
  circle A27 centre (163.044, 44.2083) radius 2
  circle A28 centre (169.566, 44.2083) radius 2
  circle A29 centre (176.088, 44.2083) radius 2
  circle A30 centre (182.61, 44.2083) radius 2
  circle A31 centre (189.132, 44.2083) radius 2
  circle A32 centre (195.654, 44.2083) radius 2
  circle A33 centre (202.176, 44.2083) radius 2
  line L10 (150, 49.2083) -> (202.176, 49.2083)
  line L11 (150, 39.2083) -> (202.176, 39.2083)
  line L12 (202.176, 44.2083) -> (207.176, 44.2083)
  arc A34 (202.176, 39.2083) -> (202.176, 49.2083) centre (202.176, 44.2083) ccw
  dimension "d69" = 6.522
  dimension "d70" = 6.522
  dimension "d71" = 6.522
  dimension "d72" = 6.522
  dimension "d73" = 6.522
  dimension "d74" = 6.522
  dimension "d75" = 6.522
  dimension "d76" = 6.522
  dimension "d77" = 4
  dimension "d78" = 4
  dimension "d79" = 4
  dimension "d80" = 4
  dimension "d81" = 4
  dimension "d82" = 4
  dimension "d83" = 4
  dimension "d84" = 4
  dimension "d85" = 5
  constraint coincident A16.centre A25.centre
  constraint horizontal L2
  constraint parallel L2 L3
  constraint parallel L2 L4
  constraint parallel L4 L5
  constraint parallel L5 L6
  constraint parallel L6 L7
  constraint parallel L6 L8
  constraint parallel L6 L9
  constraint coincident L2.end L3.start
  constraint coincident L3.end L4.start
  constraint coincident L4.end L5.start
  constraint coincident L5.end L6.start
  constraint coincident L6.end L7.start
  constraint coincident L7.end L8.start
  constraint coincident L8.end L9.start
  constraint coincident L9.end A33.centre
  constraint coincident A25.end L1.start
  constraint tangent A25 L10
  constraint coincident L0.end A25.start
  constraint tangent A25 L11
  constraint parallel L9 L12
  constraint coincident L12.end A34
  measures "d69" distance of A16.centre L2.end
  measures "d70" distance of L2.end L3.end
  measures "d71" distance of L3.end L4.end
  measures "d72" distance of L4.end L5.end
  measures "d73" distance of L5.end L6.end
  measures "d74" distance of L6.end L7.end
  measures "d75" distance of L7.end L8.end
  measures "d76" distance of L8.end L9.end
  measures "d77" diameter of A26
  measures "d78" diameter of A27
  measures "d79" diameter of A28
  measures "d80" diameter of A29
  measures "d81" diameter of A30
  measures "d82" diameter of A31
  measures "d83" diameter of A32
  measures "d84" diameter of A33
  measures "d85" distance of L9.end L12.end
extrude "Extrude20" cut sketch "Sketch19" against normal blind 10 contours A25 L3 L4 L5 L6 L7 L8 L9 A26 A27 A28 A29 A30 A31 A32 A33 L10 L12 A34 | A25 L3 L4 L5 L6 L7 L8 L9 A26 A27 A28 A29 A30 A31 A32 A33 L11 L12 A34 | A25 L2 A26 | A25 L2 A26 bodies 51
extrude "Extrude21" add sketch "Sketch19" against normal blind 10 separate body contours A25 L3 L4 L5 L6 L7 L8 L9 A26 A27 A28 A29 A30 A31 A32 A33 L10 L12 A34 | A25 L3 L4 L5 L6 L7 L8 L9 A26 A27 A28 A29 A30 A31 A32 A33 L11 L12 A34 makes body 52
combine "Combine7" operation add target body 51 tool bodies 52
copy_body "CopyPasteBodies18" bodies 51 makes body 53
move_body "Move32" bodies 53 to x (1, 0, 0) y (0, 1, 0) z (0, 0, 1) at (-96, 0, 0)
move_body "Align24" bodies 53 to x (1, 0, 0) y (0, 1, 0) z (0, 0, 1) at (6, 0, 0)
copy_body "CopyPasteBodies19" bodies 24 makes body 54
move_body "Move33" bodies 54 to x (1, 0, 0) y (0, 1, 0) z (0, 0, 1) at (-25, -45, -60)
move_body "Align25" bodies 54 to x (1, 0, 0) y (0, 1, 0) z (0, 0, 1) at (0, -0.7917, 1.3023)
move_body "Align26" bodies 54 to x (1, 0, 0) y (0, 1, 0) z (0, 0, 1) at (15, 0, 0)
extrude "Extrude22" add 1 faces at (20, 43.1049, -201.539) along direction (1, 0, 0) blind 20 separate body on bodies 54 makes body 55
combine "Combine8" operation add target body 55 tool bodies 54
copy_body "CopyPasteBodies20" bodies 25 makes body 56
move_body "Move34" bodies 56 to x (1, 0, 0) y (0, 1, 0) z (0, 0, 1) at (85, 0, 0)
move_body "Align27" bodies 56 to x (1, 0, 0) y (0, 1, 0) z (0, 0, 1) at (0, -45.7917, -58.6977)
move_body "Align28" bodies 56 to x (1, 0, 0) y (0, 1, 0) z (0, 0, 1) at (-75, 0, 0)
copy_body "CopyPasteBodies21" bodies 50 makes body 57
move_body "Move35" bodies 57 to x (1, 0, 0) y (0, 1, 0) z (0, 0, 1) at (0, 0, -210)
move_body "Align29" bodies 57 to x (1, 0, 0) y (0, 1, 0) z (0, 0, 1) at (0, -45.7917, 14.3457)
move_body "Move36" bodies 57 to x (1, 0, 0) y (0, 0, -1) z (0, 1, 0) at (0, 246.3843, -157.9677)
copy_body "CopyPasteBodies22" bodies 35 makes body 58
move_body "Move37" bodies 58 to x (1, 0, 0) y (0, 1, 0) z (0, 0, 1) at (-25, 35, 0)
move_body "Align30" bodies 58 to x (1, 0, 0) y (0, 1, 0) z (0, 0, 1) at (0, 4.25, 0)
move_body "Move38" bodies 58 to x (-1, 0, 0) y (0, -1, 0) z (0, 0, 1) at (-170, 88.4167, 0)
move_body "Align31" bodies 58 to x (1, 0, 0) y (0, 1, 0) z (0, 0, 1) at (35, 0, 0)
extrude "Extrude23" cut 1 faces at (-140, 45.3117, -142.8412) along direction (1, 0, 0) blind 60 on bodies 58 bodies 58
move_body "Move39" bodies 34 to x (1, 0, 0) y (0, 1, 0) z (0, 0, 1) at (-110, 40, 0)
move_body "Align32" bodies 34 to x (1, 0, 0) y (0, 1, 0) z (0, 0, 1) at (0, -0.75, 0)
move_body "Align33" bodies 34 to x (1, 0, 0) y (0, 1, 0) z (0, 0, 1) at (15, 0, 0)
copy_body "CopyPasteBodies23" bodies 58 34 makes body 59 makes body 60
move_body "Move40" bodies 59 60 to x (1, 0, 0) y (0, 1, 0) z (0, 0, 1) at (0, 0, 65)
move_body "Align34" bodies 59 to x (1, 0, 0) y (0, 1, 0) z (0, 0, 1) at (0, 0, 0.2174)
move_body "Align35" bodies 60 to x (1, 0, 0) y (0, 1, 0) z (0, 0, 1) at (0, 0, 0.2174)
copy_body "CopyPasteBodies24" bodies 60 59 makes body 61 makes body 62
move_body "Move41" bodies 61 62 to x (1, 0, 0) y (0, 1, 0) z (0, 0, 1) at (0, 0, 72)
move_body "Align36" bodies 62 to x (1, 0, 0) y (0, 1, 0) z (0, 0, 1) at (0, 0, -0.2609)
move_body "Align37" bodies 61 to x (1, 0, 0) y (0, 1, 0) z (0, 0, 1) at (0, 0, -0.2609)
copy_body "CopyPasteBodies25" bodies 62 60 61 59 58 34 makes body 63 makes body 64 makes body 65 makes body 66 makes body 67 makes body 68
move_body "Move42" bodies 63 64 65 66 67 68 to x (-1, 0, 0) y (0, -1, 0) z (0, 0, 1) at (-44, 88.4167, 0)
move_body "Align38" bodies 67 to x (1, 0, 0) y (0, 1, 0) z (0, 0, 1) at (4, 0, 0)
move_body "Align39" bodies 66 to x (1, 0, 0) y (0, 1, 0) z (0, 0, 1) at (4, 0, 0)
move_body "Align40" bodies 63 to x (1, 0, 0) y (0, 1, 0) z (0, 0, 1) at (4, 0, 0)
move_body "Move43" bodies 68 to x (1, 0, 0) y (0, 1, 0) z (0, 0, 1) at (4, 0, 0)
move_body "Move44" bodies 65 to x (1, 0, 0) y (0, 1, 0) z (0, 0, 1) at (4, 0, 0)
move_body "Move45" bodies 64 to x (1, 0, 0) y (0, 1, 0) z (0, 0, 1) at (4, 0, 0)
extrude "Extrude24" add 1 faces at (30, 3.8549, -142.8412) along direction (1, 0, 0) blind 20 on bodies 35 bodies 35
delete_body "RemoveBody1" bodies 22
named bodies: "Груз", "Контейнер", "Контейнер (1)"
